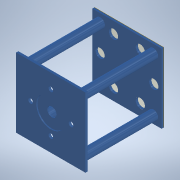
# Autodesk Inventor part: mega troque motor flange for nmrv-40
Saved by Autodesk Inventor 2020 (Build 240168000, 168)
## iProperties
Created: 2020-08-02
Part Number: mega troque motor flange for nmrv-40
Material: Generic
Document SubType Name: Modeling
Designer: Vikki
Density: 1 g/cm^3
Appearance: Flaked Satin - Blue
Author: Vikki
Autodesk Inventor part; units mm, degrees
ref_plane "YZ Plane" through (0, 0, 0) normal (1, 0, 0) x (0, 1, 0)
ref_plane "XZ Plane" through (0, 0, 0) normal (0, 1, 0) x (-1, 0, 0)
ref_plane "Work Plane1" through (0, 0, 0) normal (0, 0, 1) x (1, 0, 0)
sketch "Sketch1" plane through (0, 0, 0) normal (0, 0, 1) x (1, 0, 0)
  line L0 (-30, -30) -> (30, -30)
  line L1 (30, -30) -> (30, 30)
  line L2 (30, 30) -> (-30, 30)
  line L3 (-30, 30) -> (-30, -30)
  line L4 (-30, -30) -> (30, 30) construction
  line L5 (30, -30) -> (-30, 30) construction
  circle A0 centre (-11.6, 20.0918) radius 4 projected
  circle A1 centre (11.6, 20.0918) radius 4 projected
  circle A2 centre (-23.2, 0) radius 4 projected
  circle A3 centre (23.2, 0) radius 4 projected
  circle A4 centre (11.6, -20.0918) radius 4 projected
  circle A5 centre (-11.6, -20.0918) radius 4 projected
  point P0 (0, 0)
  point P1 (-9.5215, -21.2918)
  dimension "d0" = 60
  constraints: 12 end point, 2 midpoint, 2 parallel, 2 perpendicular, 1 horizontal, 1 other
  measures "d0" distance of L1.end L2.end
extrude "Extrusion1" add sketch "Sketch1" along normal blind 2
sketch "Sketch2" plane through (0, 0, 2) normal (0, 0, 1) x (1, 0, 0)
  line L0 (22.981, -22.981) -> (-22.981, -22.981) construction
  line L1 (-22.981, -22.981) -> (-22.981, 22.981) construction
  line L2 (-22.981, 22.981) -> (22.981, 22.981) construction
  line L3 (22.981, 22.981) -> (22.981, -22.981) construction
  line L4 (22.981, -22.981) -> (-22.981, 22.981) construction
  line L5 (-22.981, -22.981) -> (22.981, 22.981) construction
  circle A0 centre (0, 0) radius 32.5 construction
  circle A1 centre (-22.981, -22.981) radius 4
  circle A2 centre (22.981, -22.981) radius 4
  circle A3 centre (22.981, 22.981) radius 4
  circle A4 centre (-22.981, 22.981) radius 4
  dimension "d4" = 65
  dimension "d5" = 8
  dimension "d8" = 360
  constraints: 12 end point, 4 centre point, 2 coincident, 2 midpoint, 2 parallel, 2 perpendicular, 1 horizontal, 12 other
  measures "d5" diameter of A1
ref_plane "Work Plane2" through (-12.5, -12.5, 66.8) normal (0, 0, -1) x (0, 1, 0)
extrude "Extrusion2" add sketch "Sketch2" along normal up to surface (64.8 mm away)
sketch "Sketch3" plane through (-22.981, -22.981, 66.8) normal (0, 0, 1) x (1, 0, 0)
  line L0 (-7.019, -7.019) -> (52.981, -7.019) projected
  line L1 (52.981, -7.019) -> (52.981, 52.981) projected
  line L2 (-7.019, 52.981) -> (-7.019, -7.019) projected
  line L3 (52.981, 52.981) -> (-7.019, 52.981) projected
  circle A0 centre (5.481, 22.981) radius 2 projected
  circle A1 centre (22.981, 40.481) radius 2 projected
  circle A2 centre (40.481, 22.981) radius 2 projected
  circle A3 centre (22.981, 5.481) radius 2 projected
  arc A4 (22.0591, 26.8733) -> (26.4996, 24.8834) centre (22.981, 22.981) ccw projected
  circle A5 centre (22.981, 22.981) radius 4 projected
  point P0 (22.981, 22.981)
extrude "Extrusion3" add sketch "Sketch3" against normal blind 1
sketch "Sketch4" plane through (-30, -30, 66.8) normal (0, 0, 1) x (1, 0, 0)
  line L0 (0, 60) -> (0, 0) projected
  line L1 (0, 0) -> (60, 0) projected
  line L2 (60, 0) -> (60, 60) projected
  line L3 (60, 60) -> (0, 60) projected
  circle A0 centre (30, 30) radius 4 projected
  circle A1 centre (30, 12.5) radius 2 projected
  circle A2 centre (47.5, 30) radius 2 projected
  circle A3 centre (30, 47.5) radius 2 projected
  circle A4 centre (12.5, 30) radius 2 projected
  circle A5 centre (30, 30) radius 12.5 projected
  point P0 (30, 30)
extrude "Extrusion4" add sketch "Sketch4" along normal blind 1 contours L3 L2 L1 L0
body "Solid1"
